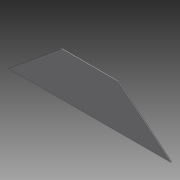
# Autodesk Inventor part: Cover_Back
Saved by Autodesk Inventor 2012 (Build 160160000, 160)
## iProperties
Created: 2012-04-27
Part Number: Cover_Back
Material: Default
Document SubType Name: Sheet Metal
Designer: Robotics
Density: 1 g/cm^3
Sheet Metal Rule: Default
Author: Robotics
Autodesk Inventor part; units mm, degrees
ref_plane "YZ Plane" through (0, 0, 0) normal (1, 0, 0) x (0, 1, 0)
ref_plane "XZ Plane" through (0, 0, 0) normal (0, 1, 0) x (-1, 0, 0)
ref_plane "XY Plane" through (0, 0, 0) normal (0, 0, 1) x (1, 0, 0)
sketch "Sketch1" plane through (0, 0, 0) normal (0, 0, 1) x (1, 0, 0)
  line L0 (-236.5375, 0) -> (236.5375, 0)
  line L1 (-82.55, 126.8984) -> (82.55, 126.8984)
  line L2 (-236.5375, 0) -> (-82.55, 126.8984)
  line L3 (236.5375, 0) -> (82.55, 126.8984)
  point P0 (0, 0)
  point P1 (0, 0)
  point P2 (0, 126.8984)
  dimension "d0" = 473.075
  dimension "d1" = 165.1
  dimension "d2" = 126.8984
  measures "d0" distance of L0.start L0.end
  measures "d1" distance of L1.start L1.end
  measures "d2" distance between parallel lines of L0 L1
extrude "Plate1" add sketch "Sketch1" along normal blind 3.048
equation "\"BendRadius\" = Thickness"
equation "\"BendReliefWidth\" = Thickness"
equation "\"BendReliefDepth\" = 0.5 * Thickness"
equation "\"CornerReliefSize\" = 4 * Thickness"
equation "\"MinimumRemnant\" = 2 * Thickness"
equation "\"TransitionRadius\" = BendRadius"
equation "\"JacobiRadiusSize\" = BendRadius"
equation "\"GapSize\" = Thickness"
equation "\"d3\" = BendRadius"
equation "\"Thickness\" = 3.048"
body "Solid1"
